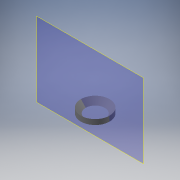
# Autodesk Inventor part: JarCollar
Saved by Autodesk Inventor 2019 (Build 230136000, 136)
## iProperties
Created: 2018-12-15
Part Number: JarCollar
Material: Generic
Document SubType Name: Modeling
Designer: assman
Density: 1 g/cm^3
Appearance: Default
Author: assman
Autodesk Inventor part; units mm, degrees
ref_plane "YZ Plane" through (0, 0, 0) normal (1, 0, 0) x (0, 1, 0)
ref_plane "XZ Plane" through (0, 0, 0) normal (0, 1, 0) x (-1, 0, 0)
ref_plane "XY Plane" through (0, 0, 0) normal (0, 0, 1) x (1, 0, 0)
ref_plane "Work Plane1" through (125.5278, 24.2206, 177.7913) normal (0, 0, -1) x (-1, 0, 0)
sketch "Sketch1" plane through (125.5278, 24.2206, 177.7913) normal (0, 0, -1) x (-1, 0, 0)
  line L0 (92, -34.5335) -> (82, -45.3253)
  line L1 (92, -45.3253) -> (92, -34.5335)
  line L2 (62, -53.3253) -> (62, 5.8556) construction
  line L3 (82, -45.3253) -> (92, -45.3253) construction
  line L4 (82, -45.3253) -> (92, -45.3253) construction
  line L5 (82, -45.3253) -> (92, -45.3253)
  point P0 (125.5278, -24.2206)
  point P1 (42, -45.3253)
  dimension "d0" = 10
  constraints: 12 end point, 2 collinear, 2 vertical, 3 other
  measures "d0" distance of L0.end L1.start
revolve "Revolution1" add sketch "Sketch1" angle 360 about axis through (63.5278, -29.1046, 177.7913) along (0, 1, 0)
body "Solid1"
